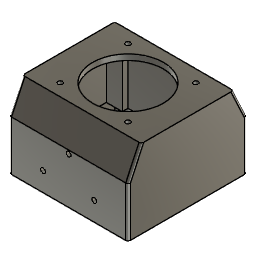
digiObscura Camera_Body (Autodesk Fusion 360 design; units mm, degrees)
Autodesk Fusion 360 part; units mm, degrees
sketch "Sketch12" plane through (0, 0, 81.6) normal (0, 0, 1) x (1, 0, 0)
  line L0 (-52, -40.3423) -> (52, -40.3423)
  line L1 (52, -40.3423) -> (52, 40.3423)
  line L2 (52, 40.3423) -> (-52, 40.3423)
  line L3 (-52, 40.3423) -> (-52, -40.3423)
  circle A0 centre (0, 0) radius 31
  line L4 (0, 52) -> (0, -52) construction
  line L5 (-52, 0) -> (52, 0) construction
  line L6 (0, 0) -> (-29.6985, -29.6985) construction
  circle A1 centre (-29.6985, -29.6985) radius 2.1
  circle A2 centre (29.6985, -29.6985) radius 2.1
  circle A3 centre (-29.6985, 29.6985) radius 2.1
  circle A4 centre (29.6985, 29.6985) radius 2.1
  dimension "d1" = 62
  dimension "d2" = 45
  dimension "d3" = 4.2
  dimension "d4" = 42
  constraint coincident A0.centre L6.start
  constraint perpendicular L2 L4
  constraint midpoint L3 L5.start
  constraint midpoint L1 L5.end
  constraint coincident L6 A1.centre
  constraint symmetric L4 A1 A2
  constraint symmetric L5 A1 A3
  constraint symmetric L5 A2 A4
  constraint coincident L6.end A1.centre
  constraint coincident A0.centre L4
  measures "d1" diameter of A0
  measures "d2" angle of L5 L6
  measures "d3" diameter of A1
  measures "d4" distance of A0.centre L6.end
ref_plane "WorkPlane2" through (-46.5, -38.5, 81.6) normal (0, 0, 1) x (1, 0, 0)
sketch "Sketch1" plane through (0, 0, 81.6) normal (0, 0, 1) x (1, 0, 0)
  line L0 (52, -52) -> (-52, -52)
  line L1 (-52, -52) -> (-52, 52)
  line L2 (-52, 52) -> (52, 52)
  line L3 (52, 52) -> (52, -52)
  line L4 (52, -52) -> (-52, 52) construction
  line L5 (-52, -52) -> (52, 52) construction
  dimension "d22" = 104
  dimension "d23" = 104
  constraint perpendicular L0 L1
  constraint parallel L0 L2
  constraint parallel L1 L3
  constraint horizontal L0
  constraint coincident L4 origin
  constraint coincident L5 origin
  measures "d22" distance of L0.start L0.end
  measures "d23" distance of L0.start L2.end
extrude "Extrude1" add sketch "Sketch1" against normal blind 68.6
sketch "Sketch2" plane through (0, 0, 13) normal (0, 0, -1) x (-1, 0, 0)
  line L0 (52, -52) -> (52, 52)
  line L1 (52, 52) -> (-52, 52)
  line L2 (-52, 52) -> (-52, -52)
  line L3 (-52, -52) -> (52, -52)
  line L4 (50.5, -50.5) -> (-50.5, -50.5)
  line L5 (-50.5, -50.5) -> (-50.5, 50.5)
  line L6 (-50.5, 50.5) -> (50.5, 50.5)
  line L7 (50.5, 50.5) -> (50.5, -50.5)
  line L8 (50.5, -50.5) -> (-50.5, 50.5) construction
  line L9 (-50.5, -50.5) -> (50.5, 50.5) construction
  dimension "d26" = 101
  dimension "d27" = 101
  constraint perpendicular L4 L5
  constraint parallel L4 L6
  constraint parallel L5 L7
  constraint horizontal L4
  constraint coincident L8 origin
  constraint coincident L9 origin
  measures "d26" distance of L4.start L4.end
  measures "d27" distance of L4.start L6.end
extrude "Extrude2" cut sketch "Sketch2" against normal blind 1.6 contours L4 L5 L6 L7
sketch "Sketch3" plane through (0, 0, 14.6) normal (0, 0, -1) x (-1, 0, 0)
  line L0 (50.5, 50.5) -> (-50.5, 50.5)
  line L1 (-50.5, 50.5) -> (-50.5, -50.5)
  line L2 (-50.5, -50.5) -> (50.5, -50.5)
  line L3 (50.5, -50.5) -> (50.5, 50.5)
  line L4 (47, -47) -> (-47, -47)
  line L5 (-47, -47) -> (-47, 47)
  line L6 (-47, 47) -> (47, 47)
  line L7 (47, 47) -> (47, -47)
  line L8 (47, -47) -> (-47, 47) construction
  line L9 (-47, -47) -> (47, 47) construction
  circle A0 centre (-47, -47) radius 4
  line L10 (-52, 0) -> (52, 0) construction
  line L11 (0, 52) -> (0, -52) construction
  circle A1 centre (47, -47) radius 4
  circle A2 centre (-47, 47) radius 4
  circle A3 centre (47, 47) radius 4
  dimension "d30" = 94
  dimension "d31" = 94
  dimension "d32" = 8
  constraint perpendicular L4 L5
  constraint parallel L4 L6
  constraint parallel L5 L7
  constraint horizontal L4
  constraint coincident L8 origin
  constraint coincident L9 origin
  constraint coincident L4.end L5.start
  constraint perpendicular L7 L10
  constraint perpendicular L2 L11
  constraint symmetric A0 L11 A1
  constraint symmetric A0 L10 A2
  constraint symmetric L10 A1 A3
  measures "d30" distance of L4.start L4.end
  measures "d31" distance of L4.start L6.end
  measures "d32" diameter of A0
extrude "Extrude3" cut sketch "Sketch3" against normal blind 12.6 contours L4 L5 L6 L7 A0 A1 A2 A3
sketch "Sketch4" plane through (0, 0, 27.2) normal (0, 0, -1) x (-1, 0, 0)
  arc A0 (-47, 43) -> (-43, 47) centre (-47, 47) ccw
  line L0 (-47, 43) -> (-47, -43)
  arc A1 (-43, -47) -> (-47, -43) centre (-47, -47) ccw
  line L1 (-43, -47) -> (43, -47)
  arc A2 (47, -43) -> (43, -47) centre (47, -47) ccw
  line L2 (47, -43) -> (47, 43)
  arc A3 (43, 47) -> (47, 43) centre (47, 47) ccw
  line L3 (43, 47) -> (-43, 47)
  line L4 (50.5, -39) -> (-50.5, -39)
  line L5 (-50.5, -39) -> (-50.5, 39)
  line L6 (-50.5, 39) -> (50.5, 39)
  line L7 (50.5, 39) -> (50.5, -39)
  line L8 (50.5, -39) -> (-50.5, 39) construction
  line L9 (-50.5, -39) -> (50.5, 39) construction
  dimension "d35" = 101
  dimension "d36" = 78
  constraint perpendicular L4 L5
  constraint parallel L4 L6
  constraint parallel L5 L7
  constraint horizontal L4
  constraint coincident L8 origin
  constraint coincident L9 origin
  measures "d35" distance of L4.start L4.end
  measures "d36" distance of L4.start L6.end
extrude "Extrude4" cut sketch "Sketch4" along normal blind 65 contours L0 L2 L4 L6 | L0 L4 L5 L6 | L2 L4 L6 L7
sketch "Sketch5" plane through (0, 0, 27.2) normal (0, 0, -1) x (-1, 0, 0)
  line L0 (-47, -39) -> (-47, -43)
  arc A0 (-43, -47) -> (-47, -43) centre (-47, -47) ccw
  line L1 (-43, -47) -> (43, -47)
  arc A1 (47, -43) -> (43, -47) centre (47, -47) ccw
  line L2 (47, -43) -> (47, -39)
  line L3 (47, -39) -> (50.5, -39)
  line L4 (50.5, -39) -> (50.5, 39)
  line L5 (50.5, 39) -> (47, 39)
  line L6 (47, 39) -> (47, 43)
  arc A2 (43, 47) -> (47, 43) centre (47, 47) ccw
  line L7 (43, 47) -> (-43, 47)
  arc A3 (-47, 43) -> (-43, 47) centre (-47, 47) ccw
  line L8 (-47, 43) -> (-47, 39)
  line L9 (-50.5, 39) -> (-50.5, -39)
  line L10 (-50.5, -39) -> (-47, -39)
  line L11 (35, -35) -> (-35, -35)
  line L12 (-35, -35) -> (-35, 35)
  line L13 (-35, 35) -> (35, 35)
  line L14 (35, 35) -> (35, -35)
  line L15 (35, -35) -> (-35, 35) construction
  line L16 (-35, -35) -> (35, 35) construction
  line L17 (49, -30) -> (-49, -30)
  line L18 (-49, -30) -> (-49, 30)
  line L19 (-49, 30) -> (49, 30)
  line L20 (49, 30) -> (49, -30)
  line L21 (49, -30) -> (-49, 30) construction
  line L22 (-49, -30) -> (49, 30) construction
  line L23 (-47, 39) -> (-50.5, 39)
  dimension "d39" = 98
  dimension "d40" = 60
  dimension "d41" = 70
  dimension "d42" = 70
  constraint perpendicular L11 L12
  constraint parallel L11 L13
  constraint parallel L12 L14
  constraint horizontal L11
  constraint coincident L15 origin
  constraint coincident L16 origin
  constraint perpendicular L17 L18
  constraint parallel L17 L19
  constraint parallel L18 L20
  constraint horizontal L17
  constraint coincident L21 origin
  constraint coincident L22 origin
  measures "d39" distance of L17.start L17.end
  measures "d40" distance of L17.start L19.end
  measures "d41" distance of L11.start L13.end
  measures "d42" distance of L12.end L13.end
extrude "Extrude5" cut sketch "Sketch5" against normal up to surface (49.4 mm away) contours L11 L12 L14 L17 | L12 L14 L17 L19 | L14 L17 L19 L20 | L12 L17 L18 L19 | L12 L13 L14 L19
chamfer "Chamfer1" distance 25 angle 25 1 edges at (0, 52, 81.6) measured on face at (-17.3333, 52, 58.7333)
chamfer "Chamfer2" distance 25 angle 25 1 edges at (0, -52, 81.6) measured on face at (17.3333, -52, 58.7333)
extrude "Extrude6" cut sketch "Sketch12" against normal through all contours A0 | A1 | A2 | A3 | A4
sketch "Sketch6" plane through (0, 0, 27.2) normal (0, 0, -1) x (-1, 0, 0)
  line L0 (-35, -35) -> (-35, -30)
  line L1 (-35, -30) -> (-49, -30)
  line L2 (-49, -30) -> (-49, 30)
  line L3 (-49, 30) -> (-35, 30)
  line L4 (-35, 30) -> (-35, 35)
  line L5 (-35, 35) -> (35, 35)
  line L6 (35, 35) -> (35, 30)
  line L7 (35, 30) -> (49, 30)
  line L8 (49, 30) -> (49, -30)
  line L9 (49, -30) -> (35, -30)
  line L10 (35, -30) -> (35, -35)
  line L11 (35, -35) -> (-35, -35)
  line L12 (-47, -39) -> (-47, -43)
  arc A0 (-43, -47) -> (-47, -43) centre (-47, -47) ccw
  line L13 (-43, -47) -> (43, -47)
  arc A1 (47, -43) -> (43, -47) centre (47, -47) ccw
  line L14 (47, -43) -> (47, -39)
  line L15 (47, -39) -> (50.5, -39)
  line L16 (50.5, -39) -> (50.5, 39)
  line L17 (50.5, 39) -> (47, 39)
  line L18 (47, 39) -> (47, 43)
  arc A2 (43, 47) -> (47, 43) centre (47, 47) ccw
  line L19 (43, 47) -> (-43, 47)
  arc A3 (-47, 43) -> (-43, 47) centre (-47, 47) ccw
  line L20 (-47, 43) -> (-47, 39)
  line L21 (-50.5, 39) -> (-50.5, -39)
  line L22 (-50.5, -39) -> (-47, -39)
  line L23 (0, 50) -> (0, -51.9143) construction
  line L24 (-55, 0) -> (55, 0) construction
  circle A4 centre (-46.5, 35.5) radius 2.1
  circle A5 centre (46.5, 35.5) radius 2.1
  circle A6 centre (-46.5, -35.5) radius 2.1
  circle A7 centre (46.5, -35.5) radius 2.1
  line L25 (-47, 39) -> (-50.5, 39)
  dimension "d77" = 4.2
  dimension "d117" = 35.5
  dimension "d118" = 46.5
  constraint perpendicular L13 L23
  constraint perpendicular L16 L24
  constraint symmetric L23 A4 A5
  constraint symmetric L24 A4 A6
  constraint symmetric L24 A5 A7
  constraint coincident origin L23
  measures "d77" diameter of A4
  measures "d117" distance of L24 A4.centre
  measures "d118" distance of L23 A4.centre
extrude "Extrude7" cut sketch "Sketch6" against normal blind 8 contours A4 | A5 | A6 | A7
sketch "Sketch7" plane through (0, 0, 14.6) normal (0, 0, -1) x (-1, 0, 0)
  line L0 (-47, 39) -> (-47, 43)
  arc A0 (-47, 43) -> (-43, 47) centre (-47, 47) ccw
  line L1 (-43, 47) -> (43, 47)
  arc A1 (43, 47) -> (47, 43) centre (47, 47) ccw
  line L2 (47, 43) -> (47, 39)
  line L3 (50.5, 39) -> (50.5, 50.5)
  line L4 (50.5, 50.5) -> (-50.5, 50.5)
  line L5 (-50.5, 50.5) -> (-50.5, 39)
  line L6 (0, 52) -> (0, -53) construction
  line L7 (-53, 0) -> (55, 0) construction
  circle A2 centre (-47, 47) radius 2.1
  circle A3 centre (47, 47) radius 2.1
  circle A4 centre (-47, -47) radius 2.1
  circle A5 centre (47, -47) radius 2.1
  line L8 (-50.5, 39) -> (-47, 39)
  line L9 (47, 39) -> (50.5, 39)
  dimension "d80" = 4.2
  constraint perpendicular L4 L6
  constraint perpendicular L6 L7
  constraint concentric A0 A2
  constraint symmetric L6 A2 A3
  constraint symmetric L7 A2 A4
  constraint symmetric L7 A3 A5
  measures "d80" diameter of A2
extrude "Extrude8" cut sketch "Sketch7" against normal blind 8 contours A2 | A3 | A4 | A5
fillet "Fillet1" radius 2 4 edges at (-52, 52, 34.8) (-52, 46.1712, 69.1) (-52, -52, 34.8) (-52, -46.1712, 69.1)
fillet "Fillet2" radius 2 4 edges at (52, 46.1712, 69.1) (52, 52, 34.8) (52, -46.1712, 69.1) (52, -52, 34.8)
fillet "Fillet3" radius 1 4 edges at (-50.5, 50.5, 13.8) (50.5, 50.5, 13.8) (50.5, -50.5, 13.8) (-50.5, -50.5, 13.8)
sketch "Sketch8" plane through (0, 47, 0) normal (0, -1, 0) x (1, 0, 0)
  line L0 (-43, 14.6) -> (43, 14.6)
  line L1 (43, 14.6) -> (43, 27.2)
  line L2 (43, 27.2) -> (-43, 27.2)
  line L3 (-43, 27.2) -> (-43, 14.6)
  circle A0 centre (-31.828, 20.7) radius 5.25
  line L4 (-31.828, 14.6) -> (-31.828, 27.2) construction
  dimension "d86" = 10.5
  dimension "d5" = 6.5
  constraint coincident L0 L4.start
  constraint coincident L2 L4.end
  constraint perpendicular L2 L4
  constraint coincident A0.centre L4
  measures "d86" diameter of A0
  measures "d5" distance of A0.centre L4.end
extrude "Extrude9" cut sketch "Sketch8" against normal blind 3 contours A0
sketch "Sketch9" plane through (0, 50, 0) normal (0, -1, 0) x (1, 0, 0)
  circle A0 centre (-31.828, 20.7) radius 3.65
  circle A1 centre (-31.828, 20.7) radius 5.25
  dimension "d89" = 7.3
  constraint coincident A0.centre A1.centre
  measures "d89" diameter of A0
extrude "Extrude10" cut sketch "Sketch9" against normal blind 8 contours A0
sketch "Sketch10" plane through (0, -52, 0) normal (0, -1, 0) x (1, 0, 0)
  line L0 (50, 13) -> (50, 56.6)
  line L1 (50, 56.6) -> (-50, 56.6)
  line L2 (-50, 56.6) -> (-50, 13)
  line L3 (-50, 13) -> (50, 13)
  circle A0 centre (0, 31) radius 22.5 construction
  circle A1 centre (0, 53.5) radius 2.1
  circle A2 centre (22.4552, 29.5809) radius 2.1
  circle A3 centre (-22.4654, 29.7532) radius 2.1
  dimension "d92" = 4.2
  dimension "d93" = 4.2
  dimension "d94" = 4.2
  dimension "d95" = 45
  constraint coincident A0 A1.centre
  constraint coincident A0 A2.centre
  constraint coincident A0 A3.centre
  measures "d92" diameter of A3
  measures "d93" diameter of A2
  measures "d94" diameter of A1
  measures "d95" diameter of A0
extrude "Extrude11" cut sketch "Sketch10" against normal blind 8 contours A1 | A2 | A3
sketch "Sketch11" plane through (-52, 0, 0) normal (-1, 0, 0) x (0, 0, 1)
  line L0 (56.1566, -50) -> (81.6, -38.1356)
  line L1 (81.6, -38.1356) -> (81.6, 38.1356)
  line L2 (81.6, 38.1356) -> (56.1566, 50)
  line L3 (56.1566, 50) -> (13, 50)
  line L4 (13, 50) -> (13, -50)
  line L5 (13, -50) -> (56.1566, -50)
  line L6 (0.3, 38) -> (14.3, 38)
  line L7 (14.3, 38) -> (14.3, 11)
  line L8 (14.3, 11) -> (0.3, 11)
  line L9 (0.3, 11) -> (0.3, 38)
  point P0 (13, 52)
  dimension "d112" = 14
  dimension "d113" = 1.3
  dimension "d114" = 41
  constraint horizontal L6
  constraint vertical L7
  constraint horizontal L8
  constraint vertical L9
  measures "d112" distance of L6 P0
  measures "d113" distance of L4 L7
  measures "d114" distance of L8 P0
extrude "Extrude12" cut sketch "Sketch11" against normal blind 2 contours L4 L6 L7 L8
equation "d33 = -11 mm - 1.6 mm"
equation "d117 = ( 71 / 2 ) * 1 mm"
equation "d118 = ( 93 / 2 ) * 1 mm"
equation "d6 = -55 mm - 12 mm - 1.6 mm"
